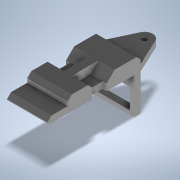
# Autodesk Inventor part: PIEZA_3D_1EX
Saved by Autodesk Inventor 2021 (Build 250183000, 183)
## iProperties
Created: 2021-02-09
Part Number: PIEZA_3D_1EX
Material: Generic
Document SubType Name: Modeling
Designer: aby_2
Density: 1 g/cm^3
Appearance: Copper - Polished
Author: aby_2
Autodesk Inventor part; units mm, degrees
ref_plane "YZ Plane" through (0, 0, 0) normal (1, 0, 0) x (0, 1, 0)
ref_plane "XZ Plane" through (0, 0, 0) normal (0, 1, 0) x (-1, 0, 0)
ref_plane "XY Plane" through (0, 0, 0) normal (0, 0, 1) x (1, 0, 0)
sketch "Sketch1" plane through (0, 0, 0) normal (0, 1, 0) x (-1, 0, 0)
  line L0 (0, 85) -> (0, -85)
  line L1 (25, 0) -> (-25, 0)
  line L2 (0, 85) -> (25, 85)
  line L3 (25, 85) -> (25, -85)
  line L4 (25, -85) -> (-25, -85)
  line L5 (-25, -85) -> (-25, 85)
  line L6 (-25, 85) -> (0, 85)
  point P0 (0, 0)
  point P1 (0, 0)
  point P2 (0, 0)
  dimension "d1" = 50
  constraints: 14 end point, 4 perpendicular, 3 horizontal, 2 coincident, 2 midpoint, 2 vertical, 1 point on line
  measures "d1" distance of L1.start L1.end
extrude "Extrusion1" add sketch "Sketch1" along normal blind 63
sketch "Sketch2" plane through (25, 0, 85) normal (1, 0, 0) x (0, 0, -1)
  line L0 (0, 0) -> (170, 0) projected
  line L1 (170, 0) -> (170, 63) projected
  line L2 (0, 63) -> (170, 63) projected
  line L3 (0, 0) -> (0, 63) projected
  line L4 (0, 0) -> (170, 0) projected
  line L5 (0, 0) -> (0, 45)
  line L6 (0, 0) -> (0, 63) projected
  line L7 (0, 45) -> (107, 45)
  line L8 (107, 45) -> (107, 0)
  point P0 (85, 0)
  dimension "d4" = 45
  dimension "d5" = 107
  constraints: 6 end point, 2 perpendicular, 2 point on line
  measures "d4" distance of L0.start L5.end
  measures "d5" distance of L5.end L7.end
extrude "Extrusion2" cut sketch "Sketch2" against normal up to next contours L3 L7 L8 L0
sketch "Sketch3" plane through (25, 0, -22) normal (0, 0, 1) x (1, 0, 0)
  line L0 (-50, 0) -> (-50, 45) projected
  line L1 (0, 0) -> (-50, 0) projected
  line L2 (0, 45) -> (0, 0) projected
  line L3 (0, 45) -> (-50, 45) projected
  line L4 (-45, 5) -> (-5, 5)
  line L5 (-5, 30) -> (-5, 5)
  line L6 (-45, 5) -> (-45, 30)
  line L7 (-45, 30) -> (-5, 30)
  point P0 (-25, 0)
  dimension "d10" = 25
  dimension "d11" = 5
  dimension "d12" = 5
  dimension "d13" = 5
  constraints: 8 end point, 2 vertical, 1 horizontal, 1 perpendicular
  measures "d10" distance between parallel lines of L4 L7
  measures "d11" distance between parallel lines of L0 L6
  measures "d12" distance from line of point (-25, 0) L4
  measures "d13" distance between parallel lines of L2 L5
extrude "Extrusion3" cut sketch "Sketch3" against normal up to next contours L6 L7 L5 L4
sketch "Sketch4" plane through (25, 0, -85) normal (1, 0, 0) x (0, 0, -1)
  line L0 (-63, 45) -> (-63, 0) projected
  line L1 (-63, 0) -> (0, 0) projected
  line L2 (0, 0) -> (0, 63) projected
  line L3 (-170, 63) -> (0, 63) projected
  line L4 (-170, 45) -> (-170, 63) projected
  line L5 (-170, 45) -> (-63, 45) projected
  line L6 (-170, 45) -> (-165, 45)
  line L7 (-170, 45) -> (-63, 45) projected
  line L8 (-165, 45) -> (-165, 63)
  line L9 (-170, 63) -> (0, 63) projected
  line L10 (-170, 45) -> (-170, 53)
  line L11 (-170, 45) -> (-170, 63) projected
  line L12 (-170, 53) -> (-165, 53)
  line L13 (-170, 53) -> (-170, 63)
  point P0 (-85, 0)
  dimension "d16" = 5
  dimension "d20" = 8
  constraints: 10 end point, 4 point on line, 2 perpendicular, 1 vertical
  measures "d16" distance of L4.start L6.end
  measures "d20" distance of L4.start L10.end
chamfer "Chamfer1" distance 2 angle 45 1 edges at (0, 45, 85)
extrude "Extrusion4" cut sketch "Sketch4" against normal up to next contours L12 L4 L3 L8
chamfer "Chamfer2" distance 5 angle 45 1 edges at (0, 53, 85)
sketch "Sketch5" plane through (25, 0, -85) normal (1, 0, 0) x (0, 0, -1)
  line L0 (-170, 48) -> (-165, 53) projected
  line L1 (-170, 47) -> (-170, 48) projected
  line L2 (-168, 45) -> (-170, 47) projected
  line L3 (-168, 45) -> (-63, 45) projected
  line L4 (-63, 45) -> (-63, 0) projected
  line L5 (-63, 0) -> (0, 0) projected
  line L6 (0, 0) -> (0, 63) projected
  line L7 (-165, 63) -> (0, 63) projected
  line L8 (-165, 63) -> (-165, 53) projected
  line L9 (-165, 53) -> (-165, 63) projected
  line L10 (-165, 53) -> (-145, 53)
  line L11 (-145, 53) -> (-145, 63)
  point P0 (-85, 0)
  dimension "d26" = 20
  constraints: 4 end point, 1 horizontal, 1 perpendicular, 1 point on line
  measures "d26" distance of L0.end L10.end
extrude "Extrusion5" cut sketch "Sketch5" against normal up to next contours L8 L7 L11 L10
chamfer "Chamfer3" distance 5 angle 45 1 edges at (0, 63, 60)
sketch "Sketch6" plane through (25, 0, -85) normal (1, 0, 0) x (0, 0, -1)
  line L0 (-145, 58) -> (-140, 63) projected
  line L1 (-145, 58) -> (-145, 53) projected
  line L2 (-145, 53) -> (-165, 53) projected
  line L3 (-170, 48) -> (-165, 53) projected
  line L4 (-170, 47) -> (-170, 48) projected
  line L5 (-168, 45) -> (-170, 47) projected
  line L6 (-168, 45) -> (-63, 45) projected
  line L7 (-63, 45) -> (-63, 0) projected
  line L8 (-63, 0) -> (0, 0) projected
  line L9 (0, 0) -> (0, 63) projected
  line L10 (-140, 63) -> (0, 63) projected
  line L11 (-170, 47) -> (-170, 0)
  line L12 (-170, 0) -> (-40, 0)
  line L13 (-63, 0) -> (0, 0) projected
  line L14 (-170, 0) -> (-55, 0)
  line L15 (-55, 0) -> (-55, 45)
  line L16 (-55, 45) -> (0, 45)
  line L17 (0, 0) -> (0, 63) projected
  line L18 (-55, 45) -> (-55, 53)
  line L19 (-55, 53) -> (0, 53)
  line L20 (-55, 53) -> (-55, 63)
  line L21 (0, 63) -> (-140, 63) projected
  line L22 (-55, 63) -> (0, 63)
  point P0 (-85, 0)
  dimension "d32" = 130
  dimension "d33" = 115
  dimension "d34" = 8
  constraints: 18 end point, 6 point on line, 2 horizontal, 2 perpendicular, 2 vertical
  measures "d32" distance of L11.end L12.end
  measures "d33" distance of L11.end L14.end
  measures "d34" distance of L15.end L18.end
extrude "Extrusion6" cut sketch "Sketch6" against normal up to next contours L10 L9 L19 L20 | L16 L9 L8 L15
sketch "Sketch7" plane through (25, 53, -30) normal (0, 1, 0) x (1, 0, 0)
  line L0 (-50, 0) -> (-50, 55) projected
  line L1 (0, 0) -> (-50, 0) projected
  line L2 (0, 55) -> (0, 0) projected
  line L3 (-50, 55) -> (0, 55) projected
  line L4 (0, 0) -> (0, 30)
  line L5 (0, 0) -> (0, 55) projected
  line L6 (0, 30) -> (-50, 30)
  line L7 (-25, -30) -> (-25, 55)
  circle A0 centre (-25, 30) radius 4
  circle A1 centre (-25, 30) radius 10
  line L8 (0, 0) -> (-15.9346, 34.2212)
  line L9 (-50, 0) -> (-34.0654, 34.2212)
  dimension "d37" = 30
  dimension "d38" = 8
  dimension "d39" = 20
  constraints: 10 end point, 3 point on line, 2 centre point, 2 midpoint, 2 point on circle, 2 tangent, 1 coincident, 1 perpendicular
  measures "d37" distance of L1.start L4.end
  measures "d38" diameter of A0
  measures "d39" diameter of A1
extrude "Extrusion7" cut sketch "Sketch7" against normal up to next contours L0 L6 L9 | L0 L3 L7 A1 L9 L6 | L8 L6 L2 | L3 L2 L6 L8 A1 L7 | A0 L6 L7 | L7 L6 A0 | A0 L7 L6 | L7 A0 L6
chamfer "Chamfer4" distance 5 angle 45 1 edges at (0, 63, -30)
sketch "Sketch8" plane through (0, 63, 0) normal (0, 1, 0) x (1, 0, 0)
  line L0 (-25, -85) -> (25, -85) projected
  line L1 (-25, 25) -> (25, 25) projected
  line L2 (-25, 25) -> (-25, -55) projected
  line L3 (25, -55) -> (-25, -55) projected
  line L4 (25, -55) -> (25, 25) projected
  line L5 (25, -85) -> (-25, -85) projected
  line L6 (25, -85) -> (36, -85)
  line L7 (36, -85) -> (36, -5)
  line L8 (25, -55) -> (25, -30)
  line L9 (25, -55) -> (25, 25) projected
  line L10 (5, -30) -> (25, -30)
  line L11 (5, -30) -> (5, -12)
  line L12 (5, -12) -> (25, -12)
  line L13 (0, -38) -> (0, 17)
  line L14 (-5, -30) -> (-25, -30)
  line L15 (-5, -30) -> (-5, -12)
  line L16 (-5, -12) -> (-25, -12)
  point P0 (0, 0)
  dimension "d45" = 80
  dimension "d46" = 25
  dimension "d47" = 20
  dimension "d48" = 18
  constraints: 20 end point, 4 symmetric about line, 3 vertical, 2 horizontal, 2 perpendicular, 2 point on line
  measures "d45" distance of L6.end L7.end
  measures "d46" distance of L3.start L8.end
  measures "d47" distance of L10.start L8.end
  measures "d48" distance of L10.start L11.end
extrude "Extrusion8" cut sketch "Sketch8" against normal blind 10 contours L16 L15 L14 L2 | L4 L10 L11 L12
chamfer "Chamfer5" distance 10 angle 45 1 edges at (15, 63, 12)
chamfer "Chamfer6" distance 10 angle 45 1 edges at (-15, 63, 12)
sketch "Sketch9" plane through (0, 53, 0) normal (0, 1, 0) x (1, 0, 0)
  line L0 (25, -30) -> (5, -30) projected
  line L1 (25, -12) -> (25, -30) projected
  line L2 (5, -12) -> (25, -12) projected
  line L3 (5, -30) -> (5, -12) projected
  line L4 (-25, -12) -> (-5, -12) projected
  line L5 (-25, -30) -> (-25, -12) projected
  line L6 (-5, -30) -> (-25, -30) projected
  line L7 (-5, -12) -> (-5, -30) projected
  line L8 (0, 0) -> (0, -34)
  line L9 (25, -12) -> (20, -12)
  line L10 (20, -12) -> (20, -25)
  line L11 (20, -25) -> (25, -25)
  line L12 (25, -83) -> (25, 22) projected
  line L13 (-5, -12) -> (-25, -12)
  line L14 (-20, -12) -> (-20, -25)
  line L15 (-20, -25) -> (-25, -25)
  dimension "d57" = 5
  dimension "d58" = 13
  constraints: 14 end point, 3 point on line, 3 symmetric about line, 2 perpendicular, 1 vertical
  measures "d57" distance of L1.start L9.end
  measures "d58" distance of L9.end L10.end
extrude "Extrusion9" cut sketch "Sketch9" against normal up to next contours L11 L10 L2 L1 | L4 L14 L15 L5
chamfer "Chamfer7" distance 5 angle 45 4 edges at (15, 63, 30) (-15, 63, 30) (25, 49, 25) (-25, 49, 25)
body "Solid1"
